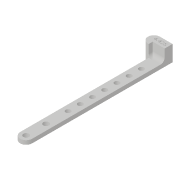
# Autodesk Inventor part: CollectorArmRear4_425long
Saved by Autodesk Inventor 2018 (Build 220112000, 112)
## iProperties
Created: 2019-02-19
Part Number: CollectorArmRear4_425long
Material: Generic
Document SubType Name: Modeling
Designer: ball
Density: 1 g/cm^3
Appearance: Default
Author: ball
Autodesk Inventor part; units mm, degrees
note: some values were not read from the file. Chosen so that the rebuilt part matches the saved one: direction of "Emboss1".
ref_plane "YZ Plane" through (0, 0, 0) normal (1, 0, 0) x (0, 1, 0)
ref_plane "XZ Plane" through (0, 0, 0) normal (0, 1, 0) x (-1, 0, 0)
ref_plane "XY Plane" through (0, 0, 0) normal (0, 0, 1) x (1, 0, 0)
sketch "Sketch1" plane through (0, 0, 0) normal (0, 1, 0) x (-1, 0, 0)
  line L0 (0, 0) -> (10.16, 0)
  line L1 (9.525, 9.6012) -> (9.525, 112.395)
  line L2 (0, 112.395) -> (0, 0)
  circle A0 centre (4.7625, 112.395) radius 2.2479
  circle A1 centre (4.7625, 96.393) radius 2.2479
  circle A2 centre (4.7625, 78.8416) radius 1.9685
  arc A3 (10.16, 0) -> (10.16, 9.6012) centre (10.16, 4.8006) ccw
  line L3 (10.16, 9.6012) -> (9.525, 9.6012)
  circle A4 centre (4.7625, 69.0626) radius 1.9685
  circle A5 centre (4.7625, 59.2836) radius 1.9685
  circle A6 centre (4.7625, 49.5046) radius 1.9685
  circle A7 centre (4.7625, 39.7256) radius 1.9685
  circle A8 centre (4.7625, 29.9466) radius 1.9685
  circle A9 centre (4.7625, 20.1676) radius 1.9685
  arc A10 (9.525, 112.395) -> (0, 112.395) centre (4.7625, 112.4455) ccw
  dimension "d0" = 9.525
  dimension "d4" = 4.4958
  dimension "d5" = 4.4958
  dimension "d6" = 16.002
  dimension "d7" = 3.937
  dimension "d8" = 17.5514
  dimension "d16" = 4.8006
  dimension "d17" = 10.16
  dimension "d18" = 112.395
  dimension "d21" = 9.779
  dimension "d27" = 4.7628
  dimension "d28" = 0
  dimension "d29" = 0
  constraints: 11 centre point, 8 end point, 4 point on circle, 2 perpendicular, 1 coincident, 1 horizontal, 1 parallel, 1 vertical, 12 other
  measures "d0" distance of L2.start L1.end
  measures "d4" diameter of A0
  measures "d5" diameter of A1
  measures "d6" distance of A1.centre A0.centre
  measures "d7" diameter of A2
  measures "d8" distance of A2.centre A1.centre
  measures "d16" distance from line of L0 point (10.16, 4.801)
  measures "d17" distance from line of L2 point (10.16, 4.801)
  measures "d18" distance from line of L0 A0.centre
  measures "d21" distance of A2.centre A4.centre
  measures "d27" radius of A10
  measures "d28" vertical distance of L1.end A0.centre
  measures "d29" vertical distance of L2.start A0.centre
extrude "Extrusion1" add sketch "Sketch1" along normal blind 3.175
sketch "Sketch2" plane through (0, 3.175, 0) normal (0, 1, 0) x (1, 0, 0)
  line L0 (-9.525, -9.6012) -> (-9.525, -6.35)
  line L1 (-9.525, -6.35) -> (0, -6.35)
  line L2 (0, -112.395) -> (0, 0) projected
  line L3 (0, -6.35) -> (0, 0)
  arc A0 (-10.16, 0) -> (-10.16, -9.6012) centre (-10.16, -4.8006) ccw projected
  arc A1 (-10.16, 0) -> (-10.239, -9.6012) centre (-10.1597, -4.8009) ccw
  line L4 (-10.16, -9.6012) -> (-9.525, -9.6012) projected
  line L5 (-9.525, -9.6012) -> (-10.16, -9.6012)
  line L6 (0, 0) -> (-10.16, 0) projected
  line L7 (-10.16, 0) -> (0, 0)
  constraints: 10 end point, 3 point on circle, 2 perpendicular, 1 centre point, 1 collinear, 1 horizontal, 1 vertical
extrude "Extrusion2" add sketch "Sketch2" along normal blind 9.525
fillet "Fillet1" radius 3.175 2 edges at (-4.7625, 3.175, 6.35) (-9.525, 3.175, 7.9756)
sketch "Sketch5" plane through (0, 12.7, 0) normal (0, 1, 0) x (1, 0, 0)
  line L0 (-11.1912, 0.0281) -> (-1.5184, 0.0281) construction
  line L1 (-1.5184, 0.0281) -> (-1.5184, -6.3829) construction
  line L2 (-1.5184, -6.3829) -> (-11.1912, -6.3829) construction
  line L3 (-11.1912, -6.3829) -> (-11.1912, 0.0281) construction
  line L4 (-9.1953, -3.8525) -> (-9.5391, -3.8525)
  line L5 (-9.5391, -3.8525) -> (-9.5391, -4.4515)
  line L6 (-9.5391, -4.4515) -> (-10.1545, -4.4515)
  line L7 (-10.1545, -4.4515) -> (-10.1545, -3.8525)
  line L8 (-10.1545, -3.8525) -> (-11.2742, -3.8525)
  line L9 (-11.2742, -3.8525) -> (-11.2742, -3.3791)
  line L10 (-11.2742, -3.3791) -> (-10.1751, -1.9053)
  line L11 (-10.1751, -1.9053) -> (-9.5391, -1.9053)
  line L12 (-9.5391, -1.9053) -> (-9.5391, -3.3956)
  line L13 (-9.5391, -3.3956) -> (-9.1953, -3.3956)
  line L14 (-9.1953, -3.3956) -> (-9.1953, -3.8525)
  line L15 (-10.1545, -3.3956) -> (-10.1545, -2.5311)
  line L16 (-10.1545, -2.5311) -> (-10.7988, -3.3956)
  line L17 (-10.7988, -3.3956) -> (-10.1545, -3.3956)
  line L18 (-8.2793, -4.4453) -> (-8.8824, -4.4453)
  line L19 (-8.8824, -4.4453) -> (-8.8824, -3.7743)
  line L20 (-8.8824, -3.7743) -> (-8.2793, -3.7743)
  line L21 (-8.2793, -3.7743) -> (-8.2793, -4.4453)
  line L22 (-5.8793, -3.8525) -> (-6.2231, -3.8525)
  line L23 (-6.2231, -3.8525) -> (-6.2231, -4.4515)
  line L24 (-6.2231, -4.4515) -> (-6.8385, -4.4515)
  line L25 (-6.8385, -4.4515) -> (-6.8385, -3.8525)
  line L26 (-6.8385, -3.8525) -> (-7.9582, -3.8525)
  line L27 (-7.9582, -3.8525) -> (-7.9582, -3.3791)
  line L28 (-7.9582, -3.3791) -> (-6.8591, -1.9053)
  line L29 (-6.8591, -1.9053) -> (-6.2231, -1.9053)
  line L30 (-6.2231, -1.9053) -> (-6.2231, -3.3956)
  line L31 (-6.2231, -3.3956) -> (-5.8793, -3.3956)
  line L32 (-5.8793, -3.3956) -> (-5.8793, -3.8525)
  line L33 (-6.8385, -3.3956) -> (-6.8385, -2.5311)
  line L34 (-6.8385, -2.5311) -> (-7.4828, -3.3956)
  line L35 (-7.4828, -3.3956) -> (-6.8385, -3.3956)
  line L36 (-3.6851, -4.4453) -> (-5.552, -4.4453)
  line L37 (-5.552, -4.4453) -> (-5.552, -4.0316)
  spline S0 degree 2 poles (-5.552, -4.0316) (-5.3153, -3.8422) (-4.9366, -3.5088) (-4.7946, -3.3585) knots 0 0 0 1 2 2 2
  spline S1 degree 2 poles (-4.7946, -3.3585) (-4.6073, -3.163) (-4.4405, -2.8645) (-4.4405, -2.7081) knots 0 0 0 1 2 2 2
  spline S2 degree 2 poles (-4.4405, -2.7081) (-4.4405, -2.5311) (-4.6525, -2.3417) (-4.8419, -2.3417) knots 0 0 0 1 2 2 2
  spline S3 degree 2 poles (-4.8419, -2.3417) (-4.9387, -2.3417) (-5.1116, -2.3891) (-5.2001, -2.4261) knots 0 0 0 1 2 2 2
  spline S4 degree 2 poles (-5.2001, -2.4261) (-5.2865, -2.4652) (-5.41, -2.5475) (-5.4409, -2.5681) knots 0 0 0 1 2 2 2
  line L38 (-5.4409, -2.5681) -> (-5.4903, -2.5681)
  line L39 (-5.4903, -2.5681) -> (-5.4903, -2.0144)
  spline S5 degree 2 poles (-5.4903, -2.0144) (-5.3833, -1.963) (-4.9263, -1.8559) (-4.7143, -1.8559) knots 0 0 0 1 2 2 2
  spline S6 degree 2 poles (-4.7143, -1.8559) (-4.2615, -1.8559) (-3.7963, -2.2594) (-3.7963, -2.6237) knots 0 0 0 1 2 2 2
  spline S7 degree 2 poles (-3.7963, -2.6237) (-3.7963, -2.8481) (-4.0083, -3.2803) (-4.2532, -3.5273) knots 0 0 0 1 2 2 2
  spline S8 degree 2 poles (-4.2532, -3.5273) (-4.4076, -3.6796) (-4.6978, -3.9163) (-4.7616, -3.9657) knots 0 0 0 1 2 2 2
  line L40 (-4.7616, -3.9657) -> (-3.6851, -3.9657)
  line L41 (-3.6851, -3.9657) -> (-3.6851, -4.4453)
  spline S9 degree 2 poles (-1.5177, -3.5849) (-1.5177, -3.7846) (-1.6535, -4.1222) (-1.7873, -4.2436) knots 0 0 0 1 2 2 2
  spline S10 degree 2 poles (-1.7873, -4.2436) (-1.9211, -4.3651) (-2.2875, -4.4989) (-2.5551, -4.4989) knots 0 0 0 1 2 2 2
  spline S11 degree 2 poles (-2.5551, -4.4989) (-2.8391, -4.4968) (-3.2467, -4.4042) (-3.3805, -4.3445) knots 0 0 0 1 2 2 2
  line L42 (-3.3805, -4.3445) -> (-3.3805, -3.7908)
  line L43 (-3.3805, -3.7908) -> (-3.3228, -3.7908)
  spline S12 degree 2 poles (-3.3228, -3.7908) (-3.2734, -3.8175) (-3.1541, -3.8875) (-3.0573, -3.9246) knots 0 0 0 1 2 2 2
  spline S13 degree 2 poles (-3.0573, -3.9246) (-2.9668, -3.9596) (-2.7794, -4.0069) (-2.6662, -4.0069) knots 0 0 0 1 2 2 2
  spline S14 degree 2 poles (-2.6662, -4.0069) (-2.5674, -4.0069) (-2.3369, -3.9575) (-2.2669, -3.8916) knots 0 0 0 1 2 2 2
  spline S15 degree 2 poles (-2.2669, -3.8916) (-2.2155, -3.8402) (-2.1578, -3.7146) (-2.1578, -3.6096) knots 0 0 0 1 2 2 2
  spline S16 degree 2 poles (-2.1578, -3.6096) (-2.1578, -3.5191) (-2.2319, -3.3915) (-2.2916, -3.3524) knots 0 0 0 1 2 2 2
  spline S17 degree 2 poles (-2.2916, -3.3524) (-2.3781, -3.2947) (-2.6251, -3.2618) (-2.7136, -3.2618) knots 0 0 0 1 2 2 2
  spline S18 degree 2 poles (-2.7136, -3.2618) (-2.8535, -3.2618) (-3.1191, -3.3071) (-3.2158, -3.3318) knots 0 0 0 1 2 2 2
  line L44 (-3.2158, -3.3318) -> (-3.2714, -3.3318)
  line L45 (-3.2714, -3.3318) -> (-3.2714, -1.9053)
  line L46 (-3.2714, -1.9053) -> (-1.5877, -1.9053)
  line L47 (-1.5877, -1.9053) -> (-1.5877, -2.3849)
  line L48 (-1.5877, -2.3849) -> (-2.6683, -2.3849)
  line L49 (-2.6683, -2.3849) -> (-2.6683, -2.8069)
  spline S19 degree 2 poles (-2.6683, -2.8069) (-2.6168, -2.8028) (-2.4748, -2.7987) (-2.4357, -2.7987) knots 0 0 0 1 2 2 2
  spline S20 degree 2 poles (-2.4357, -2.7987) (-2.2525, -2.7987) (-1.9438, -2.8728) (-1.8223, -2.9489) knots 0 0 0 1 2 2 2
  spline S21 degree 2 poles (-1.8223, -2.9489) (-1.6782, -3.0436) (-1.5177, -3.3585) (-1.5177, -3.5849) knots 0 0 0 1 2 2 2
  point P0 (0, 0)
  constraints: 2 other
emboss "Emboss1" sketch "Sketch5" operation cut depth 0.762 direction (0, -1, 0)
body "Solid1"
